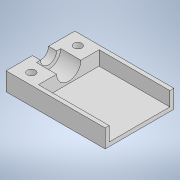
# Autodesk Inventor part: Крепление USB
Saved by Autodesk Inventor 2020 (Build 240168000, 168)
## iProperties
Created: 2021-05-10
Part Number: Крепление USB
Material: Типовые
Document SubType Name: Modeling
Designer: Антон
Density: 1 g/cm^3
Appearance: По умолчанию
Author: Антон
Autodesk Inventor part; units mm, degrees
ref_plane "YZ Plane" through (0, 0, 0) normal (1, 0, 0) x (0, 1, 0)
ref_plane "XZ Plane" through (0, 0, 0) normal (0, 1, 0) x (-1, 0, 0)
ref_plane "XY Plane" through (0, 0, 0) normal (0, 0, 1) x (1, 0, 0)
sketch "Эскиз24" plane through (0, 0, 0) normal (0, 1, 0) x (1, 0, 0)
  line L0 (0, 0) -> (24.5, 0)
  line L1 (24.5, 0) -> (24.5, 17)
  line L2 (24.5, 17) -> (0, 17)
  line L3 (0, 17) -> (0, 0)
  dimension "d124" = 24.5
  dimension "d125" = 17
  constraints: 8 end point, 2 parallel, 1 horizontal, 1 perpendicular
  measures "d124" distance of L2.end L1.end
  measures "d125" distance of L1.end L0.end
extrude "Выдавливание17" add sketch "Эскиз24" along normal blind 4.5
sketch "Эскиз25" plane through (0, 4.5, 0) normal (0, 1, 0) x (1, 0, 0)
  line L0 (24.5, 1) -> (7, 1)
  line L1 (7, 1) -> (7, 16)
  line L2 (7, 16) -> (24.5, 16)
  line L3 (24.5, 16) -> (24.5, 1)
  line L4 (24.5, 0) -> (24.5, 17) projected
  line L5 (0, 17) -> (0, 0) projected
  point P0 (24.5, 8.5)
  dimension "d128" = 15
  dimension "d129" = 17.5
  constraints: 8 end point, 2 midpoint, 2 parallel, 1 horizontal, 1 perpendicular
  measures "d128" distance of L0.end L1.end
  measures "d129" distance of L1.end L2.end
extrude "Выдавливание18" cut sketch "Эскиз25" against normal blind 3.5
sketch "Эскиз26" plane through (0, 4.5, 0) normal (0, 1, 0) x (1, 0, 0)
  line L0 (7, 1) -> (7, 16) projected
  line L1 (2, 5.5) -> (7, 5.5)
  line L2 (7, 5.5) -> (7, 11.5)
  line L3 (7, 11.5) -> (2, 11.5)
  line L4 (2, 11.5) -> (2, 5.5)
  line L5 (7, 1) -> (7, 16) projected
  point P0 (0, 0)
  point P1 (7, 8.5)
  dimension "d133" = 5
  dimension "d134" = 6
  constraints: 8 end point, 2 midpoint, 2 parallel, 1 horizontal, 1 perpendicular
  measures "d133" distance of L3.end L2.end
  measures "d134" distance of L2.end L1.end
extrude "Выдавливание19" cut sketch "Эскиз26" against normal blind 3
fillet "Сопряжение8" radius 3 2 edges at (4.5, 1.5, -11.5) (4.5, 1.5, -5.5)
sketch "Эскиз27" plane through (0, 4.5, 0) normal (0, 1, 0) x (1, 0, 0)
  line L0 (0, 6.5) -> (2, 6.5)
  line L1 (2, 6.5) -> (2, 10.5)
  line L2 (2, 10.5) -> (0, 10.5)
  line L3 (0, 10.5) -> (0, 6.5)
  line L4 (2, 5.5) -> (2, 11.5) projected
  line L5 (0, 17) -> (0, 0) projected
  point P0 (2, 8.5)
  dimension "d138" = 4
  constraints: 8 end point, 2 midpoint, 2 parallel, 1 collinear, 1 horizontal, 1 perpendicular
  measures "d138" distance of L1.end L0.end
extrude "Выдавливание20" cut sketch "Эскиз27" against normal blind 2
fillet "Сопряжение9" radius 2 2 edges at (1, 2.5, -10.5) (1, 2.5, -6.5)
sketch "Эскиз28" plane through (0, 4.5, 0) normal (0, 1, 0) x (1, 0, 0)
  line L0 (2, 11.5) -> (7, 11.5) projected
  line L1 (0, 17) -> (0, 0) projected
  line L2 (7, 11.5) -> (0, 11.5)
  line L3 (0, 11.5) -> (0, 17)
  line L4 (0, 17) -> (7, 17)
  line L5 (7, 17) -> (7, 11.5)
  line L6 (7, 5.5) -> (2, 5.5) projected
  line L7 (7, 5.5) -> (0, 5.5)
  line L8 (0, 5.5) -> (0, 0)
  line L9 (0, 0) -> (7, 0)
  line L10 (7, 0) -> (7, 5.5)
  line L11 (24.5, 17) -> (0, 17) construction
  line L12 (0, 17) -> (7, 11.5) construction
  line L13 (0, 0) -> (7, 5.5) construction
  point P0 (3.5, 14.25)
  point P1 (3.5, 2.75)
  constraints: 20 end point, 4 parallel, 2 horizontal, 2 midpoint, 2 perpendicular
hole "Отверстие6" at (3.5, 4.5, -14.25) at (3.5, 4.5, -2.75) direction (0, -1, 0) diameter 2 depth 4.5
sketch "Эскиз21" plane through (20, 0, 0.1742) normal (1, 0, 0) x (0, 0, -1)
  line L0 (0.1742, 0) -> (-5.0258, 0) projected
  line L1 (0.1742, 0) -> (0.1742, 25) projected
  line L2 (-5.0258, 0) -> (-8.7758, -17.85)
  line L3 (0.1742, 0) -> (-3.5758, -17.85)
  line L4 (-8.7758, -17.85) -> (-3.5758, -17.85)
  dimension "d103" = 17.85
  dimension "d104" = 8.95
  constraints: 6 end point, 2 parallel
  measures "d103" distance between parallel lines of L0 L4
  measures "d104" distance from line of L1 L2.end
sketch "Эскиз22" plane through (20, -17.85, 3.75) normal (0, -1, 0) x (1, 0, 0)
  line L0 (0, 0) -> (-9.1, 0)
  line L1 (-9.1, 0) -> (-9.1, 17.3)
  line L2 (-9.1, 17.3) -> (0, 17.3)
  line L3 (0, 17.3) -> (0, 0)
  line L4 (0, 5.2) -> (-9.1, 5.2) projected
  line L5 (0, 0) -> (-9.1, 0) projected
  line L6 (0, 5.2) -> (0, 0) projected
  line L7 (0, 0) -> (-9.1, 0) projected
  line L8 (-9.1, 0) -> (-9.1, 5.2) projected
  line L9 (0, 5.2) -> (-9.1, 5.2) projected
  point P0 (-20, -3.75)
  point P1 (0, -7.9181)
  point P2 (-9.1, -7.9181)
  point P3 (-9.1, 0)
  point P4 (-9.1, -7.9181)
  point P5 (0, -7.9181)
  point P6 (0, 0)
  point P7 (0, 4.1819)
  point P8 (-9.1, 4.1819)
  dimension "d122" = 12.1
  constraints: 8 end point, 3 collinear, 2 parallel, 1 horizontal, 1 perpendicular, 1 other
sketch "Эскиз23" plane through (40.15, -13.85, 3.75) normal (0, 1, 0) x (1, 0, 0)
  line L0 (-9.1, -17.3) -> (0, -17.3) projected
  line L1 (-4.55, -17.3) -> (-4.55, -12.6)
  point P0 (-40.15, 3.75)
  dimension "d118" = 4.7
  constraints: 2 end point, 1 midpoint, 1 vertical
  measures "d118" distance of L1.start L1.end
